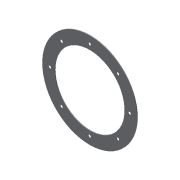
# Autodesk Inventor part: Vane_Plate
Saved by Autodesk Inventor 2022 (Build 260148000, 148)
## iProperties
Created: 2005-10-19
Part Number: Vane_Plate
Document SubType Name: Modeling
Designer: landrews
Density: 1 g/cm^3
Material: Generic
Appearance: Default
Author: landrews
Autodesk Inventor part; units mm, degrees
ref_plane "YZ Plane" through (0, 0, 0) normal (1, 0, 0) x (0, 1, 0)
ref_plane "XZ Plane" through (0, 0, 0) normal (0, 1, 0) x (-1, 0, 0)
ref_plane "XY Plane" through (0, 0, 0) normal (0, 0, 1) x (1, 0, 0)
sketch "Sketch1" plane through (0, 0, 0) normal (0, 1, 0) x (-1, 0, 0)
  line L0 (0, 7.6) -> (0, -5.7)
  line L1 (-5.7, 0) -> (7.6, 0)
  circle A0 centre (0, 0) radius 120.65
  circle A1 centre (0, 0) radius 88.9
  dimension "d0" = 31.75
  dimension "d1" = 177.8
  constraints: 4 end point, 2 centre point, 2 point on line, 1 coincident
  measures "d0" radial gap between concentric circles of A1 A0
  measures "d1" diameter of A1
extrude "Extrusion1" add sketch "Sketch1" along normal mid plane 1.905
sketch "Sketch3" plane through (0, 0, 0) normal (0, 0, 1) x (1, 0, 0)
  line L0 (-120.65, 0.9525) -> (120.65, 0.9525) projected
  line L1 (120.65, -0.9525) -> (-120.65, -0.9525) projected
  line L2 (-101.6, 0.9525) -> (-105.8749, 0.9525)
  line L3 (-105.8749, -0.9525) -> (-101.6, -0.9525)
  line L4 (-105.8749, -0.9525) -> (-98.0406, -0.9525)
  line L5 (-101.6, 0.9525) -> (-101.6, -0.9525)
  line L6 (-101.6, -0.9525) -> (-105.8749, -0.9525)
  line L7 (-88.9, -0.9525) -> (-88.9, 0.9525) projected
  line L8 (-101.6, 0.9525) -> (-105.8749, 0.9525)
  line L9 (-101.6, -0.9525) -> (-104.775, -0.9525)
  line L10 (-104.775, -0.9525) -> (-105.8749, 0.9525)
  dimension "d15" = 12.7
  dimension "d23" = 3.175
  dimension "d25" = 120
  constraints: 16 end point, 6 point on line, 2 collinear, 1 perpendicular
  measures "d15" distance from line of L7 L2.start
  measures "d23" distance of L3.end L9.end
  measures "d25" angle of L1 L10
revolve "Revolution2" cut sketch "Sketch3" angle 360 about axis through (-101.6, 0.9525, 0) along (0, -1, 0) contours L0 L5 L1 L10
pattern_circular "Circular Pattern2" count 8 over 360 about axis through (0, 0, 0) along (0, 1, 0) of "Revolution2"
body "Solid1"
